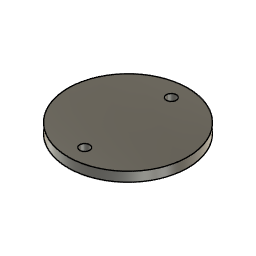
Motor Bottom Mounting Plate v1 (Autodesk Fusion 360 design; units mm, degrees)
Autodesk Fusion 360 part; units mm, degrees
sketch "Sketch1" plane through (0, 0, 0) normal (0, 0, 1) x (1, 0, 0)
  circle A0 centre (0, 0) radius 20
  dimension "d1" = 40
  constraint coincident A0.centre origin
  measures "d1" diameter of A0
extrude "Extrude1" add sketch "Sketch1" along normal blind 3.18
sketch "Sketch2" plane through (0, 0, 3.18) normal (0, 0, 1) x (-1, 0, 0)
  circle A0 centre (0, 0) radius 20
  line L0 (0, -20) -> (0, 20)
  point P0 (0, -14.5)
  point P1 (0, 14.5)
  point P2 (0, -14.5)
  point P3 (0, 14.5)
  dimension "d4" = 29
  dimension "d5" = 14.5
  constraint coincident A0 L0.start
  constraint vertical L0
  constraint coincident L0 P2
  constraint coincident L0 P3
  constraint coincident P2 P0
  constraint coincident P3 P1
  measures "d4" distance of P2 P3
  measures "d5" distance of A0.centre P2
hole "Hole1" at (0, 14.5, 3.18) at (0, -14.5, 3.18) direction (0, 0, -1) diameter 3.3 depth 25 tip angle 118
